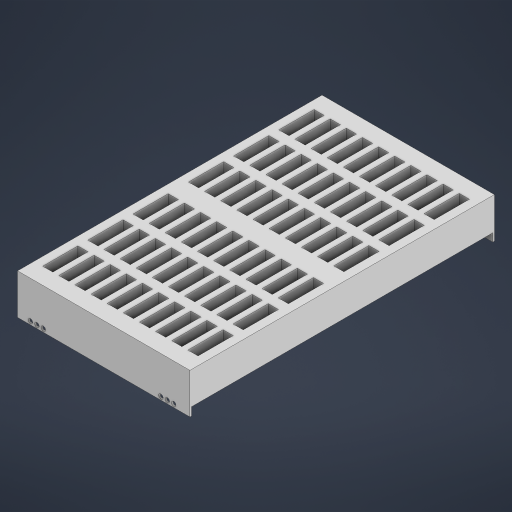
# Autodesk Inventor part: tutup
Saved by Autodesk Inventor 2024.3 (Build 283343000, 343)
## iProperties
Created: 2025-06-06
Part Number: tutup
Material: Generic
Document SubType Name: Modeling
Designer: Akbar Syihabuddin
Density: 1 g/cm^3
Appearance: Default
Author: Akbar Syihabuddin
Autodesk Inventor part; units mm, degrees
ref_plane "YZ Plane" through (0, 0, 0) normal (1, 0, 0) x (0, 1, 0)
ref_plane "XZ Plane" through (0, 0, 0) normal (0, 1, 0) x (-1, 0, 0)
ref_plane "XY Plane" through (0, 0, 0) normal (0, 0, 1) x (1, 0, 0)
sketch "Sketch1" plane through (0, 0, 0) normal (0, 1, 0) x (-1, 0, 0)
  line L0 (-73.173, 100.2562) -> (-73.173, 110.2562)
  line L1 (33.652, 78.911) -> (33.652, 110.2562)
  line L2 (-73.173, 110.2562) -> (33.652, 110.2562)
  line L3 (33.652, 110.2562) -> (33.652, 111.2562)
  line L4 (33.652, 111.2562) -> (-73.173, 111.2562)
  line L5 (-73.173, 111.2562) -> (-73.173, 110.2562)
  line L6 (-73.173, -76.4343) -> (33.652, -76.4343)
  line L7 (-73.173, -76.4343) -> (33.652, -76.4343)
  line L8 (33.652, -76.4343) -> (33.652, -77.4343)
  line L9 (33.652, -77.4343) -> (-73.173, -77.4343)
  line L10 (-73.173, -77.4343) -> (-73.173, -76.4343)
  line L11 (-73.173, -76.4343) -> (33.652, -76.4343)
  line L12 (33.652, -76.4343) -> (33.652, 110.2562)
  line L13 (33.652, 110.2562) -> (-73.173, 110.2562)
  line L14 (-73.173, 110.2562) -> (-73.173, -76.4343)
  point P0 (0, 0)
  point P1 (76.4998, -83.089)
  dimension "d0" = 1
  dimension "d1" = 1
  constraints: 30 end point, 6 parallel, 3 horizontal, 3 perpendicular
  measures "d0" distance of L3.end L2.end
  measures "d1" distance of L7.end L8.end
extrude "Extrusion1" add sketch "Sketch1" along normal blind 20
sketch "Sketch2" plane through (0, 0, 0) normal (0, -1, 0) x (1, 0, 0)
  line L0 (73.173, -77.4343) -> (-33.652, -77.4343) projected
  line L1 (-33.652, -77.4343) -> (-33.652, 111.2562) projected
  line L2 (73.173, -77.4343) -> (-33.652, -77.4343)
  line L3 (-33.652, -77.4343) -> (-33.652, -76.4343)
  line L4 (-33.652, -76.4343) -> (73.173, -76.4343)
  line L5 (73.173, -76.4343) -> (73.173, -77.4343)
  line L6 (73.173, 111.2562) -> (-33.652, 111.2562)
  line L7 (-33.652, 111.2562) -> (-33.652, 110.2562)
  line L8 (-33.652, 110.2562) -> (73.173, 110.2562)
  line L9 (73.173, 110.2562) -> (73.173, 111.2562)
  point P0 (0, 0)
  dimension "d4" = 1
  dimension "d5" = 1
  constraints: 16 end point, 4 parallel, 3 point on line, 2 horizontal, 2 perpendicular
  measures "d4" distance of L2.end L3.end
  measures "d5" distance of L7.end L6.end
extrude "Extrusion2" add sketch "Sketch2" along normal blind 5
sketch "Sketch3" plane through (0, 0, 0) normal (0, -1, 0) x (1, 0, 0)
  line L0 (73.173, 110.2562) -> (73.173, -76.4343) projected
  line L1 (67.8852, -67.1931) -> (-28.3642, -67.1931)
  line L2 (-28.3642, -67.1931) -> (-28.3642, 101.015)
  line L3 (-28.3642, 101.015) -> (67.8852, 101.015)
  line L4 (67.8852, 101.015) -> (67.8852, -67.1931)
  point P0 (0, 0)
  point P1 (-33.652, 110.2562)
  point P2 (19.7605, 16.911)
  constraints: 8 end point, 2 parallel, 1 horizontal, 1 perpendicular
extrude "Extrusion3" cut sketch "Sketch3" against normal blind 10
sketch "Sketch4" plane through (0, 20, 0) normal (0, 1, 0) x (1, 0, 0)
  line L0 (-28.3642, 67.1931) -> (-28.3642, -101.015) projected
  line L1 (-28.3642, 67.1931) -> (-22.0507, 67.1931)
  line L2 (-22.0507, 67.1931) -> (-22.0507, 45.3655)
  line L3 (-22.0507, 45.3655) -> (-28.3642, 45.3655)
  line L4 (-28.3642, 45.3655) -> (-28.3642, 67.1931)
  line L5 (67.8852, 67.1931) -> (-28.3642, 67.1931) projected
  line L6 (-28.3642, 67.1931) -> (-28.3642, -101.015) projected
  line L7 (-28.3642, -16.911) -> (63.3432, -16.911)
  line L8 (-18.3642, 67.1931) -> (-12.0507, 67.1931)
  line L9 (-12.0507, 67.1931) -> (-12.0507, 45.3655)
  line L10 (-12.0507, 45.3655) -> (-18.3642, 45.3655)
  line L11 (-18.3642, 45.3655) -> (-18.3642, 67.1931)
  line L12 (-8.3642, 67.1931) -> (-2.0507, 67.1931)
  line L13 (-2.0507, 67.1931) -> (-2.0507, 45.3655)
  line L14 (-2.0507, 45.3655) -> (-8.3642, 45.3655)
  line L15 (-8.3642, 45.3655) -> (-8.3642, 67.1931)
  line L16 (1.6358, 67.1931) -> (7.9493, 67.1931)
  line L17 (7.9493, 67.1931) -> (7.9493, 45.3655)
  line L18 (7.9493, 45.3655) -> (1.6358, 45.3655)
  line L19 (1.6358, 45.3655) -> (1.6358, 67.1931)
  line L20 (11.6358, 67.1931) -> (17.9493, 67.1931)
  line L21 (17.9493, 67.1931) -> (17.9493, 45.3655)
  line L22 (17.9493, 45.3655) -> (11.6358, 45.3655)
  line L23 (11.6358, 45.3655) -> (11.6358, 67.1931)
  line L24 (21.6358, 67.1931) -> (27.9493, 67.1931)
  line L25 (27.9493, 67.1931) -> (27.9493, 45.3655)
  line L26 (27.9493, 45.3655) -> (21.6358, 45.3655)
  line L27 (21.6358, 45.3655) -> (21.6358, 67.1931)
  line L28 (31.6358, 67.1931) -> (37.9493, 67.1931)
  line L29 (37.9493, 67.1931) -> (37.9493, 45.3655)
  line L30 (37.9493, 45.3655) -> (31.6358, 45.3655)
  line L31 (31.6358, 45.3655) -> (31.6358, 67.1931)
  line L32 (41.6358, 67.1931) -> (47.9493, 67.1931)
  line L33 (47.9493, 67.1931) -> (47.9493, 45.3655)
  line L34 (47.9493, 45.3655) -> (41.6358, 45.3655)
  line L35 (41.6358, 45.3655) -> (41.6358, 67.1931)
  line L36 (51.6358, 67.1931) -> (57.9493, 67.1931)
  line L37 (57.9493, 67.1931) -> (57.9493, 45.3655)
  line L38 (57.9493, 45.3655) -> (51.6358, 45.3655)
  line L39 (51.6358, 45.3655) -> (51.6358, 67.1931)
  line L40 (61.6358, 67.1931) -> (67.9493, 67.1931)
  line L41 (67.9493, 67.1931) -> (67.9493, 45.3655)
  line L42 (67.9493, 45.3655) -> (61.6358, 45.3655)
  line L43 (61.6358, 45.3655) -> (61.6358, 67.1931)
  line L44 (-28.3642, 39.1931) -> (-22.0507, 39.1931)
  line L45 (-22.0507, 39.1931) -> (-22.0507, 17.3655)
  line L46 (-22.0507, 17.3655) -> (-28.3642, 17.3655)
  line L47 (-28.3642, 17.3655) -> (-28.3642, 39.1931)
  line L48 (-18.3642, 39.1931) -> (-12.0507, 39.1931)
  line L49 (-12.0507, 39.1931) -> (-12.0507, 17.3655)
  line L50 (-12.0507, 17.3655) -> (-18.3642, 17.3655)
  line L51 (-18.3642, 17.3655) -> (-18.3642, 39.1931)
  line L52 (-8.3642, 39.1931) -> (-2.0507, 39.1931)
  line L53 (-2.0507, 39.1931) -> (-2.0507, 17.3655)
  line L54 (-2.0507, 17.3655) -> (-8.3642, 17.3655)
  line L55 (-8.3642, 17.3655) -> (-8.3642, 39.1931)
  line L56 (1.6358, 39.1931) -> (7.9493, 39.1931)
  line L57 (7.9493, 39.1931) -> (7.9493, 17.3655)
  line L58 (7.9493, 17.3655) -> (1.6358, 17.3655)
  line L59 (1.6358, 17.3655) -> (1.6358, 39.1931)
  line L60 (11.6358, 39.1931) -> (17.9493, 39.1931)
  line L61 (17.9493, 39.1931) -> (17.9493, 17.3655)
  line L62 (17.9493, 17.3655) -> (11.6358, 17.3655)
  line L63 (11.6358, 17.3655) -> (11.6358, 39.1931)
  line L64 (21.6358, 39.1931) -> (27.9493, 39.1931)
  line L65 (27.9493, 39.1931) -> (27.9493, 17.3655)
  line L66 (27.9493, 17.3655) -> (21.6358, 17.3655)
  line L67 (21.6358, 17.3655) -> (21.6358, 39.1931)
  line L68 (31.6358, 39.1931) -> (37.9493, 39.1931)
  line L69 (37.9493, 39.1931) -> (37.9493, 17.3655)
  line L70 (37.9493, 17.3655) -> (31.6358, 17.3655)
  line L71 (31.6358, 17.3655) -> (31.6358, 39.1931)
  line L72 (41.6358, 39.1931) -> (47.9493, 39.1931)
  line L73 (47.9493, 39.1931) -> (47.9493, 17.3655)
  line L74 (47.9493, 17.3655) -> (41.6358, 17.3655)
  line L75 (41.6358, 17.3655) -> (41.6358, 39.1931)
  line L76 (51.6358, 39.1931) -> (57.9493, 39.1931)
  line L77 (57.9493, 39.1931) -> (57.9493, 17.3655)
  line L78 (57.9493, 17.3655) -> (51.6358, 17.3655)
  line L79 (51.6358, 17.3655) -> (51.6358, 39.1931)
  line L80 (61.6358, 39.1931) -> (67.9493, 39.1931)
  line L81 (67.9493, 39.1931) -> (67.9493, 17.3655)
  line L82 (67.9493, 17.3655) -> (61.6358, 17.3655)
  line L83 (61.6358, 17.3655) -> (61.6358, 39.1931)
  line L84 (-28.3642, 11.1931) -> (-22.0507, 11.1931)
  line L85 (-22.0507, 11.1931) -> (-22.0507, -10.6345)
  line L86 (-22.0507, -10.6345) -> (-28.3642, -10.6345)
  line L87 (-28.3642, -10.6345) -> (-28.3642, 11.1931)
  line L88 (-18.3642, 11.1931) -> (-12.0507, 11.1931)
  line L89 (-12.0507, 11.1931) -> (-12.0507, -10.6345)
  line L90 (-12.0507, -10.6345) -> (-18.3642, -10.6345)
  line L91 (-18.3642, -10.6345) -> (-18.3642, 11.1931)
  line L92 (-8.3642, 11.1931) -> (-2.0507, 11.1931)
  line L93 (-2.0507, 11.1931) -> (-2.0507, -10.6345)
  line L94 (-2.0507, -10.6345) -> (-8.3642, -10.6345)
  line L95 (-8.3642, -10.6345) -> (-8.3642, 11.1931)
  line L96 (1.6358, 11.1931) -> (7.9493, 11.1931)
  line L97 (7.9493, 11.1931) -> (7.9493, -10.6345)
  line L98 (7.9493, -10.6345) -> (1.6358, -10.6345)
  line L99 (1.6358, -10.6345) -> (1.6358, 11.1931)
  line L100 (11.6358, 11.1931) -> (17.9493, 11.1931)
  line L101 (17.9493, 11.1931) -> (17.9493, -10.6345)
  line L102 (17.9493, -10.6345) -> (11.6358, -10.6345)
  line L103 (11.6358, -10.6345) -> (11.6358, 11.1931)
  line L104 (21.6358, 11.1931) -> (27.9493, 11.1931)
  line L105 (27.9493, 11.1931) -> (27.9493, -10.6345)
  line L106 (27.9493, -10.6345) -> (21.6358, -10.6345)
  line L107 (21.6358, -10.6345) -> (21.6358, 11.1931)
  line L108 (31.6358, 11.1931) -> (37.9493, 11.1931)
  line L109 (37.9493, 11.1931) -> (37.9493, -10.6345)
  line L110 (37.9493, -10.6345) -> (31.6358, -10.6345)
  line L111 (31.6358, -10.6345) -> (31.6358, 11.1931)
  line L112 (41.6358, 11.1931) -> (47.9493, 11.1931)
  line L113 (47.9493, 11.1931) -> (47.9493, -10.6345)
  line L114 (47.9493, -10.6345) -> (41.6358, -10.6345)
  line L115 (41.6358, -10.6345) -> (41.6358, 11.1931)
  line L116 (51.6358, 11.1931) -> (57.9493, 11.1931)
  line L117 (57.9493, 11.1931) -> (57.9493, -10.6345)
  line L118 (57.9493, -10.6345) -> (51.6358, -10.6345)
  line L119 (51.6358, -10.6345) -> (51.6358, 11.1931)
  line L120 (61.6358, 11.1931) -> (67.9493, 11.1931)
  line L121 (67.9493, 11.1931) -> (67.9493, -10.6345)
  line L122 (67.9493, -10.6345) -> (61.6358, -10.6345)
  line L123 (61.6358, -10.6345) -> (61.6358, 11.1931)
  line L124 (-28.3642, -101.015) -> (-22.0507, -101.015)
  line L125 (-22.0507, -101.015) -> (-22.0507, -79.1875)
  line L126 (-22.0507, -79.1875) -> (-28.3642, -79.1875)
  line L127 (-28.3642, -79.1875) -> (-28.3642, -101.015)
  line L128 (67.8852, -101.015) -> (-28.3642, -101.015)
  line L129 (-18.3642, -101.015) -> (-12.0507, -101.015)
  line L130 (-12.0507, -101.015) -> (-12.0507, -79.1875)
  line L131 (-12.0507, -79.1875) -> (-18.3642, -79.1875)
  line L132 (-18.3642, -79.1875) -> (-18.3642, -101.015)
  line L133 (-8.3642, -101.015) -> (-2.0507, -101.015)
  line L134 (-2.0507, -101.015) -> (-2.0507, -79.1875)
  line L135 (-2.0507, -79.1875) -> (-8.3642, -79.1875)
  line L136 (-8.3642, -79.1875) -> (-8.3642, -101.015)
  line L137 (1.6358, -101.015) -> (7.9493, -101.015)
  line L138 (7.9493, -101.015) -> (7.9493, -79.1875)
  line L139 (7.9493, -79.1875) -> (1.6358, -79.1875)
  line L140 (1.6358, -79.1875) -> (1.6358, -101.015)
  line L141 (11.6358, -101.015) -> (17.9493, -101.015)
  line L142 (17.9493, -101.015) -> (17.9493, -79.1875)
  line L143 (17.9493, -79.1875) -> (11.6358, -79.1875)
  line L144 (11.6358, -79.1875) -> (11.6358, -101.015)
  line L145 (21.6358, -101.015) -> (27.9493, -101.015)
  line L146 (27.9493, -101.015) -> (27.9493, -79.1875)
  line L147 (27.9493, -79.1875) -> (21.6358, -79.1875)
  line L148 (21.6358, -79.1875) -> (21.6358, -101.015)
  line L149 (31.6358, -101.015) -> (37.9493, -101.015)
  line L150 (37.9493, -101.015) -> (37.9493, -79.1875)
  line L151 (37.9493, -79.1875) -> (31.6358, -79.1875)
  line L152 (31.6358, -79.1875) -> (31.6358, -101.015)
  line L153 (41.6358, -101.015) -> (47.9493, -101.015)
  line L154 (47.9493, -101.015) -> (47.9493, -79.1875)
  line L155 (47.9493, -79.1875) -> (41.6358, -79.1875)
  line L156 (41.6358, -79.1875) -> (41.6358, -101.015)
  line L157 (51.6358, -101.015) -> (57.9493, -101.015)
  line L158 (57.9493, -101.015) -> (57.9493, -79.1875)
  line L159 (57.9493, -79.1875) -> (51.6358, -79.1875)
  line L160 (51.6358, -79.1875) -> (51.6358, -101.015)
  line L161 (61.6358, -101.015) -> (67.9493, -101.015)
  line L162 (67.9493, -101.015) -> (67.9493, -79.1875)
  line L163 (67.9493, -79.1875) -> (61.6358, -79.1875)
  line L164 (61.6358, -79.1875) -> (61.6358, -101.015)
  line L165 (-28.3642, -73.015) -> (-22.0507, -73.015)
  line L166 (-22.0507, -73.015) -> (-22.0507, -51.1875)
  line L167 (-22.0507, -51.1875) -> (-28.3642, -51.1875)
  line L168 (-28.3642, -51.1875) -> (-28.3642, -73.015)
  line L169 (-18.3642, -73.015) -> (-12.0507, -73.015)
  line L170 (-12.0507, -73.015) -> (-12.0507, -51.1875)
  line L171 (-12.0507, -51.1875) -> (-18.3642, -51.1875)
  line L172 (-18.3642, -51.1875) -> (-18.3642, -73.015)
  line L173 (-8.3642, -73.015) -> (-2.0507, -73.015)
  line L174 (-2.0507, -73.015) -> (-2.0507, -51.1875)
  line L175 (-2.0507, -51.1875) -> (-8.3642, -51.1875)
  line L176 (-8.3642, -51.1875) -> (-8.3642, -73.015)
  line L177 (1.6358, -73.015) -> (7.9493, -73.015)
  line L178 (7.9493, -73.015) -> (7.9493, -51.1875)
  line L179 (7.9493, -51.1875) -> (1.6358, -51.1875)
  line L180 (1.6358, -51.1875) -> (1.6358, -73.015)
  line L181 (11.6358, -73.015) -> (17.9493, -73.015)
  line L182 (17.9493, -73.015) -> (17.9493, -51.1875)
  line L183 (17.9493, -51.1875) -> (11.6358, -51.1875)
  line L184 (11.6358, -51.1875) -> (11.6358, -73.015)
  line L185 (21.6358, -73.015) -> (27.9493, -73.015)
  line L186 (27.9493, -73.015) -> (27.9493, -51.1875)
  line L187 (27.9493, -51.1875) -> (21.6358, -51.1875)
  line L188 (21.6358, -51.1875) -> (21.6358, -73.015)
  line L189 (31.6358, -73.015) -> (37.9493, -73.015)
  line L190 (37.9493, -73.015) -> (37.9493, -51.1875)
  line L191 (37.9493, -51.1875) -> (31.6358, -51.1875)
  line L192 (31.6358, -51.1875) -> (31.6358, -73.015)
  line L193 (41.6358, -73.015) -> (47.9493, -73.015)
  line L194 (47.9493, -73.015) -> (47.9493, -51.1875)
  line L195 (47.9493, -51.1875) -> (41.6358, -51.1875)
  line L196 (41.6358, -51.1875) -> (41.6358, -73.015)
  line L197 (51.6358, -73.015) -> (57.9493, -73.015)
  line L198 (57.9493, -73.015) -> (57.9493, -51.1875)
  line L199 (57.9493, -51.1875) -> (51.6358, -51.1875)
  line L200 (51.6358, -51.1875) -> (51.6358, -73.015)
  line L201 (61.6358, -73.015) -> (67.9493, -73.015)
  line L202 (67.9493, -73.015) -> (67.9493, -51.1875)
  line L203 (67.9493, -51.1875) -> (61.6358, -51.1875)
  line L204 (61.6358, -51.1875) -> (61.6358, -73.015)
  line L205 (-28.3642, -45.015) -> (-22.0507, -45.015)
  line L206 (-22.0507, -45.015) -> (-22.0507, -23.1875)
  line L207 (-22.0507, -23.1875) -> (-28.3642, -23.1875)
  line L208 (-28.3642, -23.1875) -> (-28.3642, -45.015)
  line L209 (-18.3642, -45.015) -> (-12.0507, -45.015)
  line L210 (-12.0507, -45.015) -> (-12.0507, -23.1875)
  line L211 (-12.0507, -23.1875) -> (-18.3642, -23.1875)
  line L212 (-18.3642, -23.1875) -> (-18.3642, -45.015)
  line L213 (-8.3642, -45.015) -> (-2.0507, -45.015)
  line L214 (-2.0507, -45.015) -> (-2.0507, -23.1875)
  line L215 (-2.0507, -23.1875) -> (-8.3642, -23.1875)
  line L216 (-8.3642, -23.1875) -> (-8.3642, -45.015)
  line L217 (1.6358, -45.015) -> (7.9493, -45.015)
  line L218 (7.9493, -45.015) -> (7.9493, -23.1875)
  line L219 (7.9493, -23.1875) -> (1.6358, -23.1875)
  line L220 (1.6358, -23.1875) -> (1.6358, -45.015)
  line L221 (11.6358, -45.015) -> (17.9493, -45.015)
  line L222 (17.9493, -45.015) -> (17.9493, -23.1875)
  line L223 (17.9493, -23.1875) -> (11.6358, -23.1875)
  line L224 (11.6358, -23.1875) -> (11.6358, -45.015)
  line L225 (21.6358, -45.015) -> (27.9493, -45.015)
  line L226 (27.9493, -45.015) -> (27.9493, -23.1875)
  line L227 (27.9493, -23.1875) -> (21.6358, -23.1875)
  line L228 (21.6358, -23.1875) -> (21.6358, -45.015)
  line L229 (31.6358, -45.015) -> (37.9493, -45.015)
  line L230 (37.9493, -45.015) -> (37.9493, -23.1875)
  line L231 (37.9493, -23.1875) -> (31.6358, -23.1875)
  line L232 (31.6358, -23.1875) -> (31.6358, -45.015)
  line L233 (41.6358, -45.015) -> (47.9493, -45.015)
  line L234 (47.9493, -45.015) -> (47.9493, -23.1875)
  line L235 (47.9493, -23.1875) -> (41.6358, -23.1875)
  line L236 (41.6358, -23.1875) -> (41.6358, -45.015)
  line L237 (51.6358, -45.015) -> (57.9493, -45.015)
  line L238 (57.9493, -45.015) -> (57.9493, -23.1875)
  line L239 (57.9493, -23.1875) -> (51.6358, -23.1875)
  line L240 (51.6358, -23.1875) -> (51.6358, -45.015)
  line L241 (61.6358, -45.015) -> (67.9493, -45.015)
  line L242 (67.9493, -45.015) -> (67.9493, -23.1875)
  line L243 (67.9493, -23.1875) -> (61.6358, -23.1875)
  line L244 (61.6358, -23.1875) -> (61.6358, -45.015)
  point P0 (0, 0)
  point P1 (0, -33.8219)
  dimension "d12" = 10
  dimension "d15" = 28
  constraints: 482 end point, 121 symmetric about line, 36 horizontal alignment, 20 parallel, 18 collinear, 2 horizontal, 1 midpoint, 1 perpendicular, 1 vertical, 164 other
  measures "d12" distance of L2.end L9.end
  measures "d15" distance of L2.end L45.end
extrude "Extrusion4" cut sketch "Sketch4" against normal blind 10
sketch "Sketch5" plane through (-33.652, 20, 111.2562) normal (0, 0, 1) x (1, 0, 0)
  line L0 (106.825, -20) -> (0, -20) projected
  line L1 (0, -20) -> (8, -20)
  line L2 (8, -20) -> (8, -23)
  circle A0 centre (8, -23) radius 1.35
  circle A1 centre (12, -23) radius 1.35
  circle A2 centre (16, -23) radius 1.35
  line L3 (106.825, -20) -> (96.825, -20)
  line L4 (96.825, -20) -> (96.825, -23)
  circle A3 centre (96.825, -23) radius 1.35
  circle A4 centre (92.825, -23) radius 1.35
  circle A5 centre (88.825, -23) radius 1.35
  point P0 (33.652, -20)
  dimension "d20" = 8
  dimension "d21" = 3
  dimension "d22" = 2.7
  dimension "d25" = 4
  dimension "d30" = 10
  dimension "d31" = 3
  dimension "d32" = 2.7
  dimension "d35" = 4
  constraints: 8 end point, 6 centre point, 2 coincident, 2 horizontal, 2 perpendicular, 2 point on line, 8 other
  measures "d20" distance of L0.end L1.end
  measures "d21" distance of L1.end L2.end
  measures "d22" diameter of A0
  measures "d25" distance of A0.centre A1.centre
  measures "d30" distance of L0.start L3.end
  measures "d31" distance of L3.end L4.end
  measures "d32" diameter of A3
  measures "d35" distance of A3.centre A4.centre
extrude "Extrusion5" cut sketch "Sketch5" against normal blind 200
body "Solid1"
